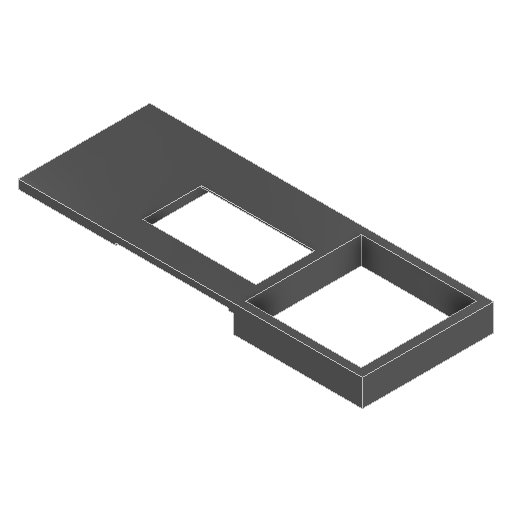
# Autodesk Inventor part: pokrywka2
Saved by Autodesk Inventor 2026.1 (Build 301233020, 233B)
## iProperties
Created: 2025-08-21
Part Number: pokrywka2
Material: Generic
Document SubType Name: Modeling
Designer: Paweł
Density: 1 g/cm^3
Appearance: Dark Gray
Author: Paweł
Autodesk Inventor part; units mm, degrees
ref_plane "YZ Plane" through (0, 0, 0) normal (1, 0, 0) x (0, 1, 0)
ref_plane "XZ Plane" through (0, 0, 0) normal (0, 1, 0) x (-1, 0, 0)
ref_plane "XY Plane" through (0, 0, 0) normal (0, 0, 1) x (1, 0, 0)
sketch "Sketch1" plane through (0, 0, 0) normal (0, 1, 0) x (-1, 0, 0)
  line L0 (-0.291, 1.3452) -> (-76.291, 1.3452)
  line L1 (-76.291, 1.3452) -> (-76.291, -27.6548)
  line L2 (-76.291, -27.6548) -> (-0.291, -27.6548)
  line L3 (-0.291, -27.6548) -> (-0.291, 1.3452)
  point P0 (0, 0)
  dimension "d0" = 76
  dimension "d1" = 29
  constraints: 8 end point, 2 parallel, 1 horizontal, 1 perpendicular
  measures "d0" distance of L2.end L1.end
  measures "d1" distance of L1.end L0.end
extrude "Extrusion1" add sketch "Sketch1" along normal blind 2
sketch "Sketch2" plane through (0, 2, 0) normal (0, 1, 0) x (1, 0, 0)
  line L0 (21.791, 4.6548) -> (46.791, 4.6548)
  line L1 (46.791, 4.6548) -> (46.791, 21.6548)
  line L2 (46.791, 21.6548) -> (21.791, 21.6548)
  line L3 (21.791, 21.6548) -> (21.791, 4.6548)
  line L4 (0.291, 27.6548) -> (0.291, -1.3452) projected
  line L5 (76.291, -1.3452) -> (76.291, 27.6548) projected
  line L6 (76.291, 27.6548) -> (0.291, 27.6548) projected
  point P0 (0, 0)
  point P1 (21.791, 13.1548)
  dimension "d4" = 25
  dimension "d5" = 17
  dimension "d10" = 29.5
  dimension "d18" = 6
  constraints: 8 end point, 2 parallel, 1 horizontal, 1 midpoint, 1 perpendicular
  measures "d4" distance of L2.end L1.end
  measures "d5" distance of L1.end L0.end
  measures "d10" distance between parallel lines of L5 L1
  measures "d18" distance between parallel lines of L6 L2
extrude "Extrusion2" cut sketch "Sketch2" against normal blind 2
sketch "Sketch3" plane through (0, 2, 0) normal (0, 1, 0) x (1, 0, 0)
  line L0 (48.791, 0.4048) -> (74.291, 0.4048)
  line L1 (74.291, 0.4048) -> (74.291, 25.9048)
  line L2 (74.291, 25.9048) -> (48.791, 25.9048)
  line L3 (48.791, 25.9048) -> (48.791, 0.4048)
  line L4 (76.291, -1.3452) -> (76.291, 27.6548) projected
  line L5 (46.791, 21.6548) -> (46.791, 4.6548) projected
  point P0 (0, 0)
  point P1 (74.291, 13.1548)
  point P2 (76.291, 13.1548)
  dimension "d8" = 25.5
  dimension "d27" = 2
  constraints: 8 end point, 2 midpoint, 2 parallel, 2 perpendicular, 1 horizontal, 1 horizontal alignment
  measures "d8" distance of L2.end L0.start
  measures "d27" distance between parallel lines of L3 L5
extrude "Extrusion3" cut sketch "Sketch3" against normal blind 2
sketch "Sketch4" plane through (0, 0, 0) normal (0, -1, 0) x (1, 0, 0)
  line L0 (74.291, -25.9048) -> (48.791, -25.9048) projected
  line L1 (48.791, -25.9048) -> (48.791, -0.4048) projected
  line L2 (48.791, -0.4048) -> (74.291, -0.4048) projected
  line L3 (74.291, -0.4048) -> (74.291, -25.9048) projected
  line L4 (46.791, -21.6548) -> (21.791, -21.6548) projected
  line L5 (21.791, -21.6548) -> (21.791, -4.6548) projected
  line L6 (21.791, -4.6548) -> (46.791, -4.6548) projected
  line L7 (46.791, -4.6548) -> (46.791, -21.6548) projected
  line L8 (76.291, 1.3452) -> (76.291, -27.6548) projected
  line L9 (0.291, 1.3452) -> (76.291, 1.3452) projected
  line L10 (0.291, -27.6548) -> (0.291, 1.3452) projected
  line L11 (76.291, -27.6548) -> (0.291, -27.6548) projected
  line L12 (21.791, -27.6548) -> (46.791, -27.6548)
  line L13 (46.791, -27.6548) -> (46.791, 1.3452)
  line L14 (46.791, 1.3452) -> (21.791, 1.3452)
  line L15 (21.791, 1.3452) -> (21.791, -27.6548)
  point P0 (0, 0)
  point P1 (46.791, -21.6548)
  point P2 (21.791, 1.3452)
  point P3 (21.791, -4.6548)
  point P4 (46.791, -4.6548)
  constraints: 8 end point, 3 point on line, 2 parallel, 1 horizontal, 1 perpendicular
extrude "Extrusion4" cut sketch "Sketch4" against normal blind 0.5 contours L13 L11 L15 L4 | L6 L15 L9 L13
sketch "Sketch9" plane through (0, 2, 0) normal (0, 1, 0) x (1, 0, 0)
  line L0 (48.791, 25.9048) -> (74.291, 25.9048) projected
  line L1 (74.291, 25.9048) -> (74.291, 0.4048) projected
  line L2 (74.291, 0.4048) -> (48.791, 0.4048) projected
  line L3 (48.791, 0.4048) -> (48.791, 25.9048) projected
  line L4 (21.791, 21.6548) -> (46.791, 21.6548) projected
  line L5 (46.791, 21.6548) -> (46.791, 4.6548) projected
  line L6 (46.791, 4.6548) -> (21.791, 4.6548) projected
  line L7 (21.791, 4.6548) -> (21.791, 21.6548) projected
  line L8 (76.291, -1.3452) -> (76.291, 27.6548) projected
  line L9 (76.291, 27.6548) -> (0.291, 27.6548) projected
  line L10 (0.291, 27.6548) -> (0.291, -1.3452) projected
  line L11 (0.291, -1.3452) -> (76.291, -1.3452) projected
  line L12 (46.791, 15.6362) -> (21.791, 15.6362)
  line L13 (21.791, 21.6548) -> (46.791, 21.6548) projected
  line L14 (21.791, 4.6548) -> (21.791, 21.6548) projected
  line L15 (46.791, 21.6548) -> (46.791, 4.6548) projected
  point P0 (0, 0)
  constraints: 2 end point, 2 point on line, 1 horizontal, 1 parallel
extrude "Extrusion9" add sketch "Sketch9" against normal blind 0.4 contours L4 L5 L12 L7
sketch "Sketch10" plane through (0, 0, 0) normal (0, -1, 0) x (1, 0, 0)
  line L0 (46.791, 1.3452) -> (46.791, -27.6548) projected
  line L1 (76.291, -27.6548) -> (46.791, -27.6548) projected
  line L2 (76.291, 1.3452) -> (76.291, -27.6548) projected
  line L3 (46.791, 1.3452) -> (76.291, 1.3452) projected
  line L4 (74.291, -25.9048) -> (48.791, -25.9048) projected
  line L5 (48.791, -25.9048) -> (48.791, -0.4048) projected
  line L6 (48.791, -0.4048) -> (74.291, -0.4048) projected
  line L7 (74.291, -0.4048) -> (74.291, -25.9048) projected
  line L8 (47.791, -26.9048) -> (75.291, -26.9048)
  line L9 (75.291, -26.9048) -> (75.291, 0.5952)
  line L10 (75.291, 0.5952) -> (47.791, 0.5952)
  line L11 (47.791, 0.5952) -> (47.791, -26.9048)
  line L12 (47.791, -26.9048) -> (47.791, -27.6548)
  line L13 (47.791, 0.5952) -> (47.791, 1.3452)
  point P0 (0, 0)
  dimension "d32" = 1
  constraints: 12 end point, 2 perpendicular, 2 point on line, 3 other
  measures "d32" distance between parallel lines of L4 L8
extrude "Extrusion10" add sketch "Sketch10" along normal blind 4 contours L3 L2 L1 L12 L8 L9 L10 L13 | L10 L9 L8 L11
sketch "Sketch13" plane through (0, 0.5, 0) normal (0, -1, 0) x (1, 0, 0)
  circle A0 centre (44.791, -1.6548) radius 1.25
  circle A1 centre (23.791, -1.6548) radius 1.25
  circle A2 centre (44.791, -24.6548) radius 1.25
  circle A3 centre (23.791, -24.6548) radius 1.25
  line L0 (44.791, -1.6548) -> (23.791, -1.6548) construction
  line L1 (46.791, -4.6548) -> (21.791, -4.6548) construction
  point P0 (0, 0)
  point P1 (51.5193, 88.3762)
  point P2 (34.291, -1.6548)
  point P3 (34.291, -4.6548)
  point P4 (21.791, 1.3452)
  dimension "d44" = 2.5
  dimension "d45" = 2.5
  dimension "d46" = 2.5
  dimension "d47" = 2.5
  dimension "d48" = 23
  dimension "d49" = 21
  dimension "d50" = 3
  constraints: 4 centre point, 3 vertical alignment, 2 end point, 2 horizontal alignment, 2 midpoint, 1 horizontal
  measures "d44" diameter of A0
  measures "d45" diameter of A1
  measures "d46" diameter of A2
  measures "d47" diameter of A3
  measures "d48" distance of A2.centre L0.start
  measures "d49" distance of L0.end L0.start
  measures "d50" vertical distance of point (21.791, 1.345) L0.end
extrude "Extrusion13" add sketch "Sketch13" along normal blind 1
sketch "Sketch14" plane through (0, 1.6, 0) normal (0, -1, 0) x (1, 0, 0)
  line L0 (46.791, -15.6362) -> (46.791, -21.6548) projected
  line L1 (46.791, -15.6362) -> (21.791, -15.6362) projected
  line L2 (21.791, -21.6548) -> (21.791, -15.6362) projected
  line L3 (46.791, -21.6548) -> (21.791, -21.6548) projected
  line L4 (46.791, -17.6362) -> (21.791, -17.6362)
  point P0 (0, 0)
  dimension "d53" = 2
  constraints: 2 end point, 2 point on line, 1 perpendicular
  measures "d53" distance between parallel lines of L1 L4
extrude "Extrusion14" cut sketch "Sketch14" against normal blind 1 contours L0 L4 L2 L1
body "Solid1"
